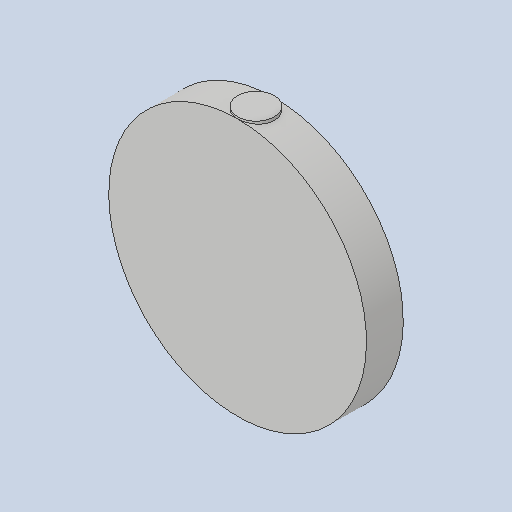
# Autodesk Inventor part: ч ASY human dummy 01
Saved by Autodesk Inventor 2025 (Build 290162010, 162A)
## iProperties
Created: 2019-08-19
Part Number: ч ASY human dummy 01
Material: Типовые
Document SubType Name: Modeling
Designer: admin
Density: 1 g/cm^3
Appearance: По умолчанию
Author: admin
Autodesk Inventor part; units mm, degrees
ref_plane "YZ Plane" through (0, 0, 0) normal (1, 0, 0) x (0, 1, 0)
ref_plane "XZ Plane" through (0, 0, 0) normal (0, 1, 0) x (-1, 0, 0)
ref_plane "XY Plane" through (0, 0, 0) normal (0, 0, 1) x (1, 0, 0)
sketch "Эскиз3" plane through (0, 0, 0) normal (0, 0, 1) x (1, 0, 0)
  circle A0 centre (0, 0) radius 70
  dimension "d1" = 140
  constraints: 1 centre point, 1 coincident
  measures "d1" diameter of A0
extrude "Выдавливание1" add sketch "Эскиз3" along normal mid plane 20
sketch "Эскиз4" plane through (0, 0, 0) normal (0, 1, 0) x (-1, 0, 0)
  circle A0 centre (0, 0) radius 10
  dimension "d4" = 20
  constraints: 1 centre point, 1 coincident
  measures "d4" diameter of A0
extrude "Выдавливание2" add sketch "Эскиз4" along normal blind 71
equation "\"d1\" = hip_diam"
equation "\"d4\" = joint_width"
equation "\"hip_diam\" = 140"
equation "\"joint_width\" = 20"
